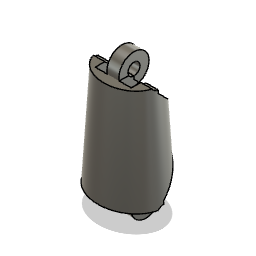
pinky finger aligned v1 (Autodesk Fusion 360 archive; units mm, degrees)
design "pinky part 2"
Autodesk Fusion 360 part; units mm, degrees
note: some values were not read from the file. Set by a fixed rule: which sketch regions a step uses.
sketch "Sketch1" plane through (0, 0, 0) normal (0, 1, 0) x (1, 0, 0)
  ellipse E0 centre (0, 0) end of major axis (6, 0) minor radius 5
  line L0 (-6, 0) -> (6, 0) construction
  line L1 (0, -5) -> (0, 5) construction
  dimension "d1" = 12
  dimension "d2" = 10
  constraint coincident E0 L0.start
  constraint coincident E0 L0.end
  constraint coincident E0 L1.start
  constraint coincident E0 L1.end
  constraint coincident E0.centre origin
  constraint horizontal L0
  measures "d1" distance of E0
ref_plane "WorkPlane1" through (0, 17, 0) normal (0, 1, 0) x (1, 0, 0)
sketch "Sketch2" plane through (0, 17, 0) normal (0, 1, 0) x (1, 0, 0)
  ellipse E0 centre (0, 0) end of major axis (5, 0) minor radius 4
  line L0 (-5, 0) -> (5, 0) construction
  line L1 (0, -4) -> (0, 4) construction
  constraint coincident E0 L0.start
  constraint coincident E0 L0.end
  constraint coincident E0 L1.start
  constraint coincident E0 L1.end
  constraint coincident E0.centre origin
  constraint horizontal L0
loft "Loft1" add profiles "Sketch1", "Sketch2" section 1 section 2 makes body 1
sketch "Sketch3" plane through (0, 0, 0) normal (1, 0, 0) x (0, 0, -1)
  line L0 (0, 0) -> (0, 1)
  line L1 (0, 1) -> (6, 7)
  line L2 (6, 7) -> (6, 0)
  line L3 (6, 0) -> (0, 0)
  line L4 (0, 17) -> (0, 16)
  line L5 (0, 16) -> (5.5, 10.5)
  line L6 (5.5, 10.5) -> (5.5, 17)
  line L7 (5.5, 17) -> (0, 17)
  dimension "d4" = 1
  constraint coincident L0.start L3.end
  constraint vertical L0
  constraint parallel L0 L2
  constraint perpendicular L0 L3
  constraint vertical L4
  constraint parallel L4 L6
  constraint perpendicular L4 L7
  measures "d4" distance of L0.start L0.end
extrude "Extrude1" cut sketch "Sketch3" along normal mid plane 16 bodies 1
sketch "Sketch4" plane through (0, 0, 0) normal (1, 0, 0) x (0, 0, -1)
  circle A0 centre (0, -0.5) radius 2.5
  circle A1 centre (0, 17.5) radius 2.5
  dimension "d7" = 5
  dimension "d8" = 5
  measures "d7" diameter of A0
  measures "d8" diameter of A1
extrude "Extrude2" add sketch "Sketch4" along normal mid plane 6 separate body makes body 2 at (2, 17.3754, -2.4969) makes body 3 at (2, -0.6246, -2.4969)
extrude "Extrude3" cut 1 faces at (-3, 15.7487, 0.1854) along direction (1, 0, 0) blind 2 on bodies 2 bodies 1 2
extrude "Extrude4" cut 1 faces at (3, 15.7487, 0.1854) along direction (-1, 0, 0) blind 2 on bodies 2 bodies 1 2
extrude "Extrude5" cut 1 faces at (-3, -1.0437, -0.4573) along direction (1, 0, 0) blind 4 on bodies 3 bodies 1 3
copy_body "CopyPasteBodies1" bodies 3 makes body 4
move_body "Move1" bodies 4 to x (1, 0, 0) y (0, 1, 0) z (0, 0, 1) at (-4, 0, 0)
sketch "Sketch5" plane through (0, 0, 0) normal (1, 0, 0) x (0, 0, -1)
  circle A0 centre (0, -0.5) radius 1
  circle A1 centre (0, 17.5) radius 1
  dimension "d17" = 2
  dimension "d18" = 2
  measures "d17" diameter of A0
  measures "d18" diameter of A1
extrude "Extrude6" cut sketch "Sketch5" along normal mid plane 20 bodies 1 2 3 4

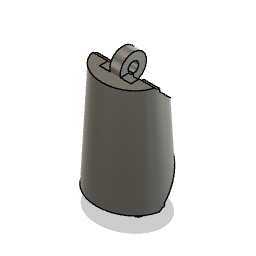
design "pinky part 3"
Autodesk Fusion 360 part; units mm, degrees
sketch "Sketch1" plane through (0, 0, 0) normal (0, 1, 0) x (1, 0, 0)
  ellipse E0 centre (0, 0) end of major axis (7, 0) minor radius 6
  line L0 (-7, 0) -> (7, 0) construction
  line L1 (0, -6) -> (0, 6) construction
  dimension "d2" = 12
  constraint coincident E0 L0.start
  constraint coincident E0 L0.end
  constraint coincident E0 L1.start
  constraint coincident E0 L1.end
  constraint coincident E0.centre origin
  constraint horizontal L0
ref_plane "WorkPlane1" through (0, 20, 0) normal (0, 1, 0) x (1, 0, 0)
sketch "Sketch2" plane through (0, 20, 0) normal (0, 1, 0) x (1, 0, 0)
  ellipse E0 centre (0, 0) end of major axis (6, 0) minor radius 5
  line L0 (-6, 0) -> (6, 0) construction
  line L1 (0, -5) -> (0, 5) construction
  dimension "d3" = 10
  constraint coincident E0 L0.start
  constraint coincident E0 L0.end
  constraint coincident E0 L1.start
  constraint coincident E0 L1.end
  constraint coincident E0.centre origin
  constraint horizontal L0
sketch "Sketch3" plane through (0, 20, 0) normal (0, 1, 0) x (1, 0, 0)
loft "Loft1" add profiles "Sketch1", "Sketch2" section 1 section 2 makes body 1
sketch "Sketch4" plane through (0, 0, 0) normal (1, 0, 0) x (0, 0, -1)
  line L0 (0, 0) -> (0, 1)
  line L1 (0, 1) -> (7, 8)
  line L2 (7, 8) -> (7, 0)
  line L3 (7, 0) -> (0, 0)
  line L4 (0, 20) -> (0, 19)
  line L5 (0, 19) -> (5.7581, 13.2325)
  line L6 (5.7581, 13.2325) -> (5.7581, 20)
  line L7 (5.7581, 20) -> (0, 20)
  point P0 (0, 20)
  constraint coincident L0.start L3.end
  constraint vertical L0
  constraint parallel L0 L2
  constraint perpendicular L0 L3
  constraint coincident P0 L4.start
  constraint vertical L4
  constraint parallel L4 L6
  constraint perpendicular L4 L7
extrude "Extrude1" cut sketch "Sketch4" along normal through all and the other way through all bodies 1
sketch "Sketch5" plane through (0, 0, 0) normal (1, 0, 0) x (0, 0, -1)
  circle A0 centre (0, -0.5) radius 2.5
  circle A1 centre (0, 20.5) radius 2.5
  dimension "d5" = 5
  dimension "d6" = 5
  measures "d5" diameter of A0
  measures "d6" diameter of A1
extrude "Extrude2" add sketch "Sketch5" along normal mid plane 6 separate body makes body 2 at (2, 20.3754, -2.4969) makes body 3 at (2, -0.6246, -2.4969)
extrude "Extrude3" cut 1 faces at (-3, 20.6214, -0.8056) along direction (1, 0, 0) blind 2 on bodies 2 bodies 1 2
extrude "Extrude4" cut 1 faces at (3, 20.6214, -0.8056) along direction (-1, 0, 0) blind 2 on bodies 2 bodies 1 2
extrude "Extrude5" cut 1 faces at (-3, -1.0437, -0.4573) along direction (1, 0, 0) blind 4 on bodies 3 bodies 1 3
copy_body "CopyPasteBodies1" bodies 3 makes body 4
move_body "Move1" bodies 4 to x (1, 0, 0) y (0, 1, 0) z (0, 0, 1) at (-4, 0, 0)
sketch "Sketch6" plane through (0, 0, 0) normal (1, 0, 0) x (0, 0, -1)
  circle A0 centre (0, -0.5) radius 1
  circle A1 centre (0, 20.5) radius 1
  dimension "d15" = 2
  dimension "d16" = 2
  measures "d15" diameter of A0
  measures "d16" diameter of A1
extrude "Extrude6" cut sketch "Sketch6" along normal through all and the other way through all bodies 1 2 3 4

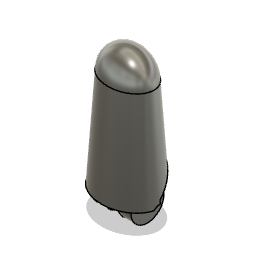
design "pinky part 1"
Autodesk Fusion 360 part; units mm, degrees
sketch "1st ellipse" plane through (0, 0, 0) normal (0, 1, 0) x (1, 0, 0)
  ellipse E0 centre (0, 0) end of major axis (5, 0) minor radius 4
  line L0 (-5, 0) -> (5, 0) construction
  line L1 (0, -4) -> (0, 4) construction
  constraint coincident E0 L0.start
  constraint coincident E0 L0.end
  constraint coincident E0 L1.start
  constraint coincident E0 L1.end
  constraint coincident E0.centre origin
  constraint horizontal L0
ref_plane "WorkPlane1" through (0, 15, 0) normal (0, 1, 0) x (1, 0, 0)
sketch "top elipse" plane through (0, 15, 0) normal (0, 1, 0) x (1, 0, 0)
  ellipse E0 centre (0, 0) end of major axis (4, 0) minor radius 3
  line L0 (-4, 0) -> (4, 0) construction
  line L1 (0, -3) -> (0, 3) construction
  constraint coincident E0 L0.start
  constraint coincident E0 L0.end
  constraint coincident E0 L1.start
  constraint coincident E0 L1.end
  constraint coincident E0.centre origin
  constraint horizontal L0
loft "Loft1" add profiles "1st ellipse", "top elipse" section 1 section 2 makes body 1
sketch "line over small elipse" plane through (0, 15, 0) normal (0, 1, 0) x (-1, 0, 0)
  ellipse E0 centre (0, 0) end of major axis (-4, 0) minor radius 3
  ellipse E1 centre (0, 0) end of major axis (-4, 0) minor radius 3
  line L0 (4, 0) -> (-4, 0) construction
  line L1 (0, 3) -> (0, -3) construction
  line L2 (0, -3) -> (0, 3)
  constraint coincident E1 L0.start
  constraint coincident E1 L0.end
  constraint coincident E1 L1.start
  constraint coincident E1 L1.end
  constraint coincident E0.centre E1.centre
  constraint horizontal L0
  constraint coincident L1.end L2.start
  constraint coincident L1.start L2.end
revolve "Revolve1" add sketch "line over small elipse" angle 360 about axis through (0, 15, 3) along (0, 0, -1) separate body contours E0 E1 L2 picked at (-0.4011, 0.9861) makes body 2
sketch "trapezium " plane through (0, 0, 0) normal (1, 0, 0) x (0, 0, -1)
  line L0 (0, 0) -> (0, 1)
  line L1 (0, 1) -> (4.5, 5.5)
  line L2 (4.5, 5.5) -> (4.5, 0)
  line L3 (4.5, 0) -> (0, 0)
  dimension "d3" = 1
  constraint coincident L0.start L3.end
  constraint vertical L0
  constraint parallel L0 L2
  constraint perpendicular L0 L3
  measures "d3" distance of L0.start L0.end
extrude "Extrude1" cut sketch "trapezium " along normal through all and the other way through all bodies 1
sketch "big circle" plane through (0, 0, 0) normal (1, 0, 0) x (0, 0, -1)
  circle A0 centre (0, -0.5) radius 2.5
  dimension "d5" = 5
  measures "d5" diameter of A0
extrude "Extrude2" add sketch "big circle" along normal mid plane 6 separate body makes body 3
extrude "Extrude3" cut 1 faces at (-3, -1.0437, -0.4573) along direction (1, 0, 0) blind 2 on bodies 3 bodies 1 3
extrude "Extrude4" cut 1 faces at (3, -1.0437, -0.4573) along direction (-1, 0, 0) blind 2 on bodies 3 bodies 1 3
sketch "small circle" plane through (-3, 0, 0) normal (1, 0, 0) x (0, 0, -1)
  line L0 (0, 1) -> (0.8508, 1.8508)
  arc A0 (0.8508, 1.8508) -> (-2.4495, 0) centre (0, -0.5) ccw
  line L1 (-2.4495, 0) -> (0, 0)
  line L2 (0, 0) -> (0, 1)
  circle A1 centre (0, -0.5) radius 1
  dimension "d12" = 2
  constraint concentric A0 A1
  measures "d12" diameter of A1
extrude "Extrude5" cut sketch "small circle" along normal mid plane 18 contours L1 L2 A1 | L1 L2 A1 bodies 1 3
sketch "Sketch7" plane through (0, 0, 0) normal (0, 0, 1) x (1, 0, 0)
sketch "Sketch8" plane through (0, 0, 0) normal (1, 0, 0) x (0, 0, -1)
extrude "Extrude6" add 1 faces at (1, -0.6739, -1.987) along direction (1, 0, 0) blind 2 on bodies 3 bodies 1 2 3
extrude "Extrude7" cut 1 faces at (-1, -2.4451, 0.4457) along direction (1, 0, 0) blind 2 on bodies 1 bodies 1
sketch "Sketch9" plane through (0, 0, 0) normal (1, 0, 0) x (0, 0, -1)
  circle A0 centre (0, -0.5) radius 2.5
  dimension "d19" = 5
  measures "d19" diameter of A0
extrude "Extrude8" add sketch "Sketch9" against normal blind 3 separate body makes body 4
extrude "Extrude9" cut 1 faces at (0, 0.1515, -0.5196) along direction (-1, 0, 0) blind 1 on bodies 4 bodies 4
extrude "Extrude10" cut sketch "small circle" along normal blind 3 contours L1 L2 A1 | L1 L2 A1 bodies 4
